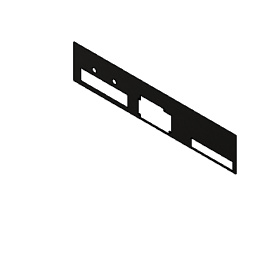
003_backing_plate (Autodesk Fusion 360 design; units mm, degrees)
Autodesk Fusion 360 part; units mm, degrees
sketch "Sketch1" plane through (0, 0, -193) normal (0, 0, -1) x (-1, 0, 0)
  arc A0 (-238.5, 15) -> (-233.5, 10) centre (-233.5, 15) ccw
  line L0 (-233.5, 10) -> (-31.5, 10)
  arc A1 (-31.5, 10) -> (-26.5, 15) centre (-31.5, 15) ccw
  line L1 (-26.5, 15) -> (-26.5, 55)
  arc A2 (-26.5, 55) -> (-31.5, 60) centre (-31.5, 55) ccw
  line L2 (-31.5, 60) -> (-233.5, 60)
  arc A3 (-233.5, 60) -> (-238.5, 55) centre (-233.5, 55) ccw
  line L3 (-238.5, 55) -> (-238.5, 15)
  arc A4 (-239, 14.5) -> (-234, 9.5) centre (-234, 14.5) ccw
  line L4 (-234, 9.5) -> (-31, 9.5)
  arc A5 (-31, 9.5) -> (-26, 14.5) centre (-31, 14.5) ccw
  line L5 (-26, 14.5) -> (-26, 55.5)
  arc A6 (-26, 55.5) -> (-31, 60.5) centre (-31, 55.5) ccw
  line L6 (-31, 60.5) -> (-234, 60.5)
  arc A7 (-234, 60.5) -> (-239, 55.5) centre (-234, 55.5) ccw
  line L7 (-239, 55.5) -> (-239, 14.5)
  line L8 (0, 140) -> (0, 0)
  line L9 (0, 0) -> (-720, 0)
  line L10 (-720, 0) -> (-720, 140)
  line L11 (-720, 140) -> (0, 140)
  line L12 (-710, 0) -> (-604, 0) construction
  line L13 (-604, 0) -> (-604, 35) construction
  line L14 (-604, 35) -> (-710, 35) construction
  line L15 (-710, 35) -> (-710, 0) construction
  line L16 (-435.408, 0) -> (-284.408, 0) construction
  line L17 (-284.408, 0) -> (-284.408, 88)
  line L18 (-284.408, 88) -> (-435.408, 88)
  line L19 (-435.408, 88) -> (-435.408, 0)
  line L20 (-603, 0) -> (-603, 36)
  line L21 (-603, 36) -> (-711, 36)
  line L22 (-711, 36) -> (-711, 0)
  circle A8 centre (-87.5, 80.5) radius 10
  circle A9 centre (-177.5, 80.5) radius 10
  line L23 (-177.5, 80.5) -> (-87.5, 80.5) construction
  line L24 (-711, 36) -> (-523, 36)
  line L25 (-523, 36) -> (-523, -2)
  line L26 (-523, -2) -> (-711, -2)
  line L27 (-711, -2) -> (-711, 36)
  line L28 (-132.5, 60.5) -> (-132.5, 80.5) construction
  line L29 (-435.408, 0) -> (-423.908, 0)
  line L30 (-423.908, 0) -> (-423.908, 12)
  line L31 (-423.908, 12) -> (-435.408, 12)
  line L32 (-435.408, 12) -> (-435.408, 0)
  line L33 (-284.408, 0) -> (-294.908, 0)
  line L34 (-294.908, 0) -> (-294.908, 12)
  line L35 (-294.908, 12) -> (-284.408, 12)
  line L36 (-284.408, 12) -> (-284.408, 0)
  line L37 (-284.408, 88) -> (-294.908, 88)
  line L38 (-294.908, 88) -> (-294.908, 68)
  line L39 (-294.908, 68) -> (-284.408, 68)
  line L40 (-284.408, 68) -> (-284.408, 88)
  line L41 (-435.408, 88) -> (-399.908, 88)
  line L42 (-399.908, 88) -> (-399.908, 78)
  line L43 (-399.908, 78) -> (-435.408, 78)
  line L44 (-435.408, 78) -> (-435.408, 88)
  line L45 (-290.908, 6) -> (-289.908, 6)
  arc A10 (-289.908, 6) -> (-289.908, 10) centre (-289.908, 8) ccw
  line L46 (-289.908, 10) -> (-290.908, 10)
  arc A11 (-290.908, 10) -> (-290.908, 6) centre (-290.908, 8) ccw
  line L47 (-290.908, 8) -> (-289.908, 8) construction
  line L48 (-290.408, 88) -> (-290.408, 72) construction
  line L49 (-290.408, 72) -> (-290.408, 8) construction
  line L50 (-290.408, 8) -> (-428.408, 8) construction
  line L51 (-428.408, 8) -> (-428.408, 82) construction
  line L52 (-290.408, 82) -> (-404.408, 82) construction
  line L53 (-404.408, 82) -> (-428.408, 82) construction
  arc A12 (-290.908, 74) -> (-290.908, 70) centre (-290.908, 72) ccw
  line L54 (-290.908, 70) -> (-289.908, 70)
  arc A13 (-289.908, 70) -> (-289.908, 74) centre (-289.908, 72) ccw
  line L55 (-290.908, 72) -> (-289.908, 72) construction
  line L56 (-289.908, 74) -> (-290.908, 74)
  arc A14 (-403.908, 80) -> (-403.908, 84) centre (-403.908, 82) ccw
  line L57 (-427.908, 10) -> (-428.908, 10)
  line L58 (-428.908, 8) -> (-427.908, 8) construction
  arc A15 (-404.908, 84) -> (-404.908, 80) centre (-404.908, 82) ccw
  line L59 (-404.908, 80) -> (-403.908, 80)
  line L60 (-404.908, 82) -> (-403.908, 82) construction
  arc A16 (-427.908, 6) -> (-427.908, 10) centre (-427.908, 8) ccw
  line L61 (-428.908, 6) -> (-427.908, 6)
  line L62 (-403.908, 84) -> (-404.908, 84)
  arc A17 (-428.908, 10) -> (-428.908, 6) centre (-428.908, 8) ccw
  line L63 (5, -5) -> (-725, -5)
  line L64 (-725, -5) -> (-725, 145)
  line L65 (-725, 145) -> (5, 145)
  line L66 (5, 145) -> (5, -5)
  point P0 (-290.408, 8)
  point P1 (-290.408, 72)
  point P2 (-404.408, 82)
  point P3 (-428.408, 8)
  dimension "d395" = 1
  dimension "d412" = 20
  dimension "d415" = 20
  dimension "d443" = 80
  dimension "d504" = 20
  dimension "d505" = 90
  dimension "d773" = 4
  dimension "d777" = 1
  dimension "d778" = 16
  dimension "d779" = 64
  dimension "d780" = 6
  dimension "d781" = 138
  dimension "d782" = 74
  dimension "d784" = 114
  dimension "d785" = 4
  dimension "d786" = 1
  dimension "d787" = 4
  dimension "d788" = 1
  dimension "d789" = 4
  dimension "d790" = 1
  dimension "d791" = 2
  dimension "d792" = 4
  dimension "d793" = 2
  dimension "d794" = 4
  dimension "d795" = 2
  dimension "d796" = 4
  dimension "d797" = 2
  dimension "d798" = 4
  dimension "d887" = -5
  constraint coincident A9.centre L23.start
  constraint coincident A8.centre L23.end
  constraint horizontal L23
  constraint horizontal L24
  constraint vertical L25
  constraint horizontal L26
  constraint vertical L27
  constraint collinear L21 L24
  constraint collinear L22 L27
  constraint midpoint L6 L28.start
  constraint midpoint L23 L28.end
  constraint vertical L28
  constraint horizontal L29
  constraint vertical L30
  constraint horizontal L31
  constraint vertical L32
  constraint coincident L16.start L19.end
  constraint horizontal L33
  constraint vertical L34
  constraint horizontal L35
  constraint vertical L36
  constraint coincident L16.end L17.start
  constraint horizontal L37
  constraint vertical L38
  constraint horizontal L39
  constraint vertical L40
  constraint coincident L17.end L18.start
  constraint horizontal L41
  constraint vertical L42
  constraint horizontal L43
  constraint vertical L44
  constraint coincident L18.end L19.start
  constraint tangent L45 A10
  constraint tangent A10 L46
  constraint parallel L45 L46
  constraint tangent L46 A11
  constraint tangent L45 A11
  constraint horizontal L47
  constraint midpoint L47 P0
  constraint coincident L18 L48.start
  constraint perpendicular L18 L48
  constraint parallel L48 L49
  constraint perpendicular L49 L50
  constraint perpendicular L31 L51
  constraint horizontal L52
  constraint coincident L48 L52.start
  constraint tangent L54 A13
  constraint tangent A13 L56
  constraint parallel L54 L56
  constraint tangent A12 L56
  constraint tangent A12 L54
  constraint horizontal L55
  constraint midpoint P1 L55
  constraint tangent A16 L61
  constraint tangent L57 A16
  constraint parallel L57 L61
  constraint tangent L57 A17
  constraint tangent L61 A17
  constraint horizontal L58
  constraint midpoint P3 L58
  constraint tangent A14 L59
  constraint tangent A14 L62
  constraint parallel L59 L62
  constraint tangent A15 L62
  constraint tangent A15 L59
  constraint horizontal L60
  constraint midpoint P2 L60
  constraint coincident P0 L49.end
  constraint coincident P3 L50.end
  constraint coincident P2 L52.end
  constraint coincident P1 L48.end
  constraint horizontal L53
  measures "d412" diameter of A8
  measures "d415" diameter of A9
  measures "d443" distance of L20 L25
  measures "d504" distance of L28.start L28.end
  measures "d505" distance of A8.centre A9.centre
  measures "d773" diameter of A10
  measures "d777" distance of A10.end L46.end
  measures "d778" distance of L48.start P1
  measures "d779" distance of P1 P0
  measures "d780" distance of L17 L48
  measures "d781" distance of P0 P3
  measures "d782" distance of P3 L51.end
  measures "d784" distance of L52.start P2
  measures "d785" diameter of A13
  measures "d786" distance of A12.start A13.end
  measures "d787" diameter of A16
  measures "d788" distance of L57.end L57.start
  measures "d789" diameter of A14
  measures "d790" distance of A14.end A15.start
  measures "d791" distance of L39 L54
  measures "d792" distance of L38 A12.centre
  measures "d793" distance of L43 L59
  measures "d794" distance of L42 A14.centre
  measures "d795" distance of L31 L57
  measures "d796" distance of L30 L58.end
  measures "d797" distance of L35 L46
  measures "d798" distance of L34 A11.centre
extrude "Extrude1" add sketch "Sketch1" against normal blind 1 contours L8 L9 L10 L11 L17 L18 L19 L21 L22 L24 L25 L27 L32 L36 L37 L40 L41 L44 | L9 L17 L33 L34 L35 L36 | L9 L19 L29 L30 L31 L32 | L17 L18 L37 L38 L39 L40 | L18 L19 L41 L42 L43 L44
ref_plane "WorkPlane1" through (0, 70, 0) normal (0, -1, 0) x (1, 0, 0)
extrude "Extrude2" add sketch "Sketch1" against normal up to surface (1 mm away) contours L9 L25 L26 L27 | L63 L64 L65 L66
equation "d792 = d785 / 2 + 2 mm"
equation "d793 = d791"
equation "d794 = d792"
equation "d795 = d791"
equation "d796 = d792"
equation "d797 = d791"
equation "d798 = d792"
